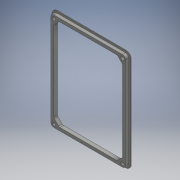
# Autodesk Inventor part: SolarPanel_CoilForm
Saved by Autodesk Inventor 2017 (Build 210142000, 142)
## iProperties
Created: 2018-05-13
Part Number: SolarPanel_CoilForm
Material: ABS Plastic
Document SubType Name: Modeling
Designer: Bradley
Density: 1.06 g/cm^3
Appearance: Smooth - Medium Gray
Author: Bradley
Autodesk Inventor part; units mm, degrees
ref_plane "YZ Plane" through (0, 0, 0) normal (1, 0, 0) x (0, 1, 0)
ref_plane "XZ Plane" through (0, 0, 0) normal (0, 1, 0) x (-1, 0, 0)
ref_plane "XY Plane" through (0, 0, 0) normal (0, 0, 1) x (1, 0, 0)
sketch "Sketch1" plane through (0, 0, 0) normal (0, 1, 0) x (-1, 0, 0)
  line L0 (33, 44) -> (-33, 44) construction
  line L1 (-33, 44) -> (-33, -44) construction
  line L2 (-33, -44) -> (33, -44) construction
  line L3 (33, -44) -> (33, 44) construction
  line L4 (33, 49) -> (-33, 49)
  line L5 (-38, 44) -> (-38, -44)
  line L6 (-33, -49) -> (33, -49)
  line L7 (38, -44) -> (38, 44)
  arc A0 (38, 44) -> (33, 49) centre (33, 44) ccw
  arc A1 (-33, 49) -> (-38, 44) centre (-33, 44) ccw
  arc A2 (-38, -44) -> (-33, -49) centre (-33, -44) ccw
  arc A3 (33, -49) -> (38, -44) centre (33, -44) ccw
  line L8 (-33, 47) -> (33, 47)
  arc A4 (36, 44) -> (33, 47) centre (33, 44) ccw
  line L9 (36, 44) -> (36, -44)
  arc A5 (33, -47) -> (36, -44) centre (33, -44) ccw
  line L10 (33, -47) -> (-33, -47)
  arc A6 (-36, -44) -> (-33, -47) centre (-33, -44) ccw
  line L11 (-36, -44) -> (-36, 44)
  arc A7 (-33, 47) -> (-36, 44) centre (-33, 44) ccw
  circle A8 centre (33, 44) radius 1.65
  circle A9 centre (33, -44) radius 1.65
  circle A10 centre (-33, -44) radius 1.65
  circle A11 centre (-33, 44) radius 1.65
  line L12 (33, 39) -> (28, 44)
  line L13 (28, 44) -> (-28, 44)
  line L14 (-28, 44) -> (-33, 39)
  line L15 (-33, 39) -> (-33, -39)
  line L16 (-33, -39) -> (-28, -44)
  line L17 (-28, -44) -> (28, -44)
  line L18 (28, -44) -> (33, -39)
  line L19 (33, -39) -> (33, 39)
  point P0 (0, 0)
  point P1 (33, 0)
  point P2 (38, 49)
  point P3 (-38, 49)
  point P4 (38, -49)
  point P5 (-38, 0)
  point P6 (0, 49)
  point P7 (0, 44)
  dimension "d0" = 76
  dimension "d1" = 98
  dimension "d2" = 5
  dimension "d3" = 2
  dimension "d4" = 3.3
  dimension "d5" = 1.35
  dimension "d6" = 1.35
  dimension "d7" = 66
  dimension "d8" = 88
  dimension "d9" = 5
  dimension "d10" = 3.5355
  constraints: 40 end point, 16 point on circle, 14 point on line, 12 centre point, 9 perpendicular, 8 tangent, 6 equal radius, 6 parallel, 5 midpoint, 4 coincident, 2 horizontal, 2 horizontal alignment, 2 vertical alignment, 7 other
  measures "d0" distance of point (38, 49) point (-38, 49)
  measures "d1" distance of point (38, -49) point (38, 49)
  measures "d2" radius of A0
  measures "d3" distance between parallel lines of L9 L7
  measures "d4" diameter of A8
  measures "d5" distance edge to line of A8 L8
  measures "d6" distance edge to line of A8 L9
  measures "d7" distance of L0.start L0.end
  measures "d8" distance of L2.end L0.start
  measures "d9" horizontal distance of L12.start L12.end
  measures "d10" distance from line of L0.start L12
extrude "Extrusion1" add sketch "Sketch1" along normal mid plane 3.5 contours A0 L7 A3 L6 A2 L5 A1 L4 | L8 A4 L9 A5 L10 A6 L11 A7
fillet "Fillet1" radius 2 8 edges at (-33, 0, -39) (-28, 0, -44) (28, 0, -44) (33, 0, -39) (33, 0, 39) (28, 0, 44) (-33, 0, 39) (-28, 0, 44)
extrude "Extrusion2" cut sketch "Sketch1" along normal blind 1.25 and the other way blind 1.75 contours A0 L7 A3 L6 A2 L5 A1 L4
body "Solid1"
